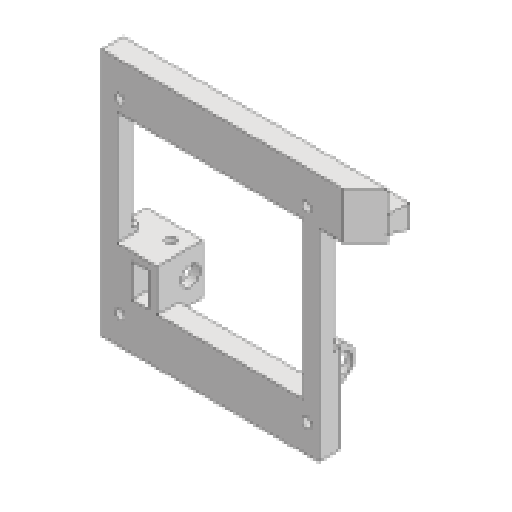
# Autodesk Inventor part: Rail_carriage_y_top_v2
Saved by Autodesk Inventor 2023 (Build 270158000, 158)
## iProperties
Created: 2022-01-11
Part Number: Rail_carriage_y_top_v2
Material: Generic
Document SubType Name: Modeling
Designer: CDT
Density: 1 g/cm^3
Appearance: Default
Author: CDT
Autodesk Inventor part; units mm, degrees
ref_plane "YZ Plane" through (0, 0, 0) normal (1, 0, 0) x (0, 1, 0)
ref_plane "XZ Plane" through (0, 0, 0) normal (0, 1, 0) x (-1, 0, 0)
sketch "Sketch1" plane through (0, 0, 0) normal (0, 0, 1) x (1, 0, 0)
  line L0 (58.7032, 31.1168) -> (-11.2968, 31.1168)
  line L1 (-11.2968, 31.1168) -> (-11.2968, -48.8832)
  line L2 (-11.2968, -48.8832) -> (58.7032, -48.8832)
  line L3 (58.7032, -48.8832) -> (58.7032, 31.1168)
  line L4 (53.7032, 16.1168) -> (-6.2968, 16.1168)
  line L5 (-6.2968, 16.1168) -> (-6.2968, -33.8832)
  line L6 (-6.2968, -33.8832) -> (53.7032, -33.8832)
  line L7 (53.7032, -33.8832) -> (53.7032, 16.1168)
  line L8 (58.7032, 31.1168) -> (73.7032, 31.1168)
  line L9 (73.7032, 31.1168) -> (73.7032, 16.1168)
  line L10 (73.7032, 16.1168) -> (58.7032, 16.1168)
  line L11 (58.7032, 16.1168) -> (58.7032, 31.1168)
  point P0 (0, 0)
  dimension "d0" = 70
  dimension "d1" = 80
  dimension "d4" = 60
  dimension "d5" = 50
  dimension "d6" = 15
  dimension "d7" = 5
  dimension "d76" = 15
  dimension "d77" = 15
  constraints: 24 end point, 6 parallel, 3 horizontal, 3 perpendicular
  measures "d0" distance of L2.end L1.end
  measures "d1" distance of L1.end L0.end
  measures "d4" distance of L6.end L5.end
  measures "d5" distance of L5.end L4.end
  measures "d6" distance between parallel lines of L0 L4
  measures "d7" distance between parallel lines of L3 L7
  measures "d76" distance of L9.end L10.end
  measures "d77" distance of L8.end L9.end
extrude "Extrusion1" add sketch "Sketch1" along normal blind 7
sketch "Sketch2" plane through (0, 0, 0) normal (0, 0, -1) x (-1, 0, 0)
  line L0 (11.2968, 23.8168) -> (-73.7032, 23.8168)
  line L1 (-73.7032, 23.8168) -> (-73.7032, 18.4168)
  line L2 (-73.7032, 18.4168) -> (11.2968, 18.4168)
  line L3 (11.2968, 18.4168) -> (11.2968, 23.8168)
  line L4 (11.2968, 31.1168) -> (11.2968, -48.8832) projected
  line L5 (-58.7032, -48.8832) -> (-58.7032, 16.1168) projected
  line L6 (-73.7032, 16.1168) -> (-73.7032, 31.1168) projected
  line L7 (-73.7032, 31.1168) -> (11.2968, 31.1168) projected
  point P0 (0, 0)
  dimension "d9" = 5.4
  dimension "d10" = 0
  dimension "d78" = 0
  dimension "d79" = 7.3
  constraints: 8 end point, 2 parallel, 1 horizontal, 1 perpendicular
  measures "d9" distance between parallel lines of L2 L0
  measures "d10" distance between parallel lines of L4 L3
  measures "d78" distance between parallel lines of L6 L1
  measures "d79" distance between parallel lines of L7 L0
extrude "Extrusion2" add sketch "Sketch2" along normal blind 5.9 draft 9.9 contours L3 L2 L1 L0
ref_plane "Work Plane1" through (-126.6696, -48.8832, -9) normal (0, 0, 1) x (1, 0, 0)
sketch "Sketch3" plane through (0, 0, 0) normal (0, 0, -1) x (-1, 0, 0)
  line L0 (11.2968, -36.3832) -> (-6.7032, -36.3832)
  line L1 (-6.7032, -36.3832) -> (-6.7032, -20.3832)
  line L2 (-6.7032, -20.3832) -> (11.2968, -20.3832)
  line L3 (11.2968, -20.3832) -> (11.2968, -36.3832)
  line L4 (11.2968, -48.8832) -> (-58.7032, -48.8832) projected
  line L5 (11.2968, 18.4168) -> (11.2968, -48.8832) projected
  line L6 (-55.7032, -33.3832) -> (-53.7032, -33.3832)
  line L7 (-53.7032, -33.3832) -> (-53.7032, -22.3832)
  line L8 (-53.7032, -22.3832) -> (-55.7032, -22.3832)
  line L9 (-55.7032, -22.3832) -> (-55.7032, -33.3832)
  line L10 (-53.7032, -33.8832) -> (6.2968, -33.8832) projected
  line L11 (-53.7032, 16.1168) -> (-53.7032, -33.8832) projected
  point P0 (0, 0)
  point P1 (-54.7032, -33.3832)
  dimension "d14" = 16
  dimension "d15" = 18
  dimension "d16" = 12.5
  dimension "d17" = 0
  dimension "d62" = 11
  dimension "d63" = 0
  dimension "d64" = 2
  dimension "d102" = 0.5
  constraints: 16 end point, 4 parallel, 2 horizontal, 2 perpendicular, 1 midpoint
  measures "d14" distance between parallel lines of L0 L2
  measures "d15" distance between parallel lines of L3 L1
  measures "d16" distance between parallel lines of L4 L0
  measures "d17" distance between parallel lines of L5 L3
  measures "d62" distance between parallel lines of L8 L6
  measures "d63" distance between parallel lines of L11 L7
  measures "d64" distance between parallel lines of L9 L11
  measures "d102" distance from line of L10 point (-54.703, -33.383)
extrude "Extrusion3" add sketch "Sketch3" along normal blind 7.5
sketch "Sketch6" plane through (0, 0, 7) normal (0, 0, 1) x (1, 0, 0)
  line L0 (-6.2968, -20.3832) -> (6.7032, -20.3832) projected
  line L1 (-11.2968, -48.8832) -> (58.7032, -48.8832) projected
  line L2 (6.7032, -20.3832) -> (-11.2968, -20.3832)
  line L3 (-11.2968, -20.3832) -> (-11.2968, -48.8832)
  line L4 (-11.2968, -48.8832) -> (6.7032, -48.8832)
  line L5 (6.7032, -48.8832) -> (6.7032, -20.3832)
  point P0 (0, 0)
  point P1 (6.7032, -48.8832)
  point P2 (-6.2968, -20.3832)
  constraints: 8 end point, 2 parallel, 1 horizontal, 1 perpendicular
extrude "Extrusion6" add sketch "Sketch6" against normal up to surface (7 mm away)
sketch "Sketch9" plane through (-11.2968, -48.8832, 7) normal (-1, 0, 0) x (0, 0, 1)
  circle A0 centre (-10.75, 20.5) radius 3.125
  line L0 (0, 80) -> (0, 0) projected
  line L1 (-7, 0) -> (0, 0) projected
  line L2 (-7, 28.5) -> (-7, 65) projected
  point P0 (-7, 48.8832)
  point P1 (-4, 28.5)
  point P2 (-7, 65)
  dimension "d44" = 6.25
  dimension "d46" = 20.5
  dimension "d65" = 3.75
  constraints: 1 centre point, 1 other
  measures "d44" diameter of A0
  measures "d46" distance from line of L1 A0.centre
extrude "Extrusion8" cut sketch "Sketch9" against normal through all
sketch "Sketch10" plane through (0, 0, -7.5) normal (0, 0, -1) x (-1, 0, 0)
  line L0 (1.4968, -23.0332) -> (-3.7032, -23.0332)
  line L1 (-3.7032, -23.0332) -> (-3.7032, -33.7332)
  line L2 (-3.7032, -33.7332) -> (1.4968, -33.7332)
  line L3 (1.4968, -33.7332) -> (1.4968, -23.0332)
  line L4 (11.2968, -20.3832) -> (-6.7032, -20.3832) projected
  line L5 (-6.7032, -36.3832) -> (11.2968, -36.3832) projected
  line L6 (-6.7032, -20.3832) -> (-6.7032, -36.3832) projected
  point P0 (0, 0)
  dimension "d49" = 5.2
  dimension "d50" = 10.7
  dimension "d51" = 2.65
  dimension "d52" = 2.65
  dimension "d53" = 3
  constraints: 8 end point, 2 parallel, 1 horizontal, 1 perpendicular
  measures "d49" distance between parallel lines of L3 L1
  measures "d50" distance between parallel lines of L2 L0
  measures "d51" distance between parallel lines of L4 L0
  measures "d52" distance between parallel lines of L5 L2
  measures "d53" distance between parallel lines of L6 L1
extrude "Extrusion9" cut sketch "Sketch10" against normal through all
sketch "Sketch11" plane through (-6.2968, -20.3832, 7) normal (0, 1, 0) x (1, 0, 0)
  circle A0 centre (8, 9.5) radius 1.5
  line L0 (10, 14.5) -> (10, 0) projected
  line L1 (-5, 14.5) -> (13, 14.5) projected
  point P0 (6.2968, 7)
  dimension "d56" = 3
  dimension "d57" = 2
  dimension "d58" = 5
  constraints: 1 centre point
  measures "d56" diameter of A0
  measures "d57" distance from line of L0 A0.centre
  measures "d58" distance from line of L1 A0.centre
extrude "Extrusion10" cut sketch "Sketch11" against normal blind 5
sketch "Sketch12" plane through (0, 0, 0) normal (0, 0, -1) x (-1, 0, 0)
  line L0 (-58.7032, -20.3832) -> (-53.7032, -20.3832)
  line L1 (-53.7032, -20.3832) -> (-53.7032, 12.1168)
  line L2 (-53.7032, 12.1168) -> (-58.7032, 12.1168)
  line L3 (-58.7032, 12.1168) -> (-58.7032, -20.3832)
  line L4 (-53.7032, -22.3832) -> (-55.7032, -22.3832) projected
  line L5 (-53.7032, 16.1168) -> (-53.7032, -22.3832) projected
  line L6 (6.2968, 16.1168) -> (-53.7032, 16.1168) projected
  line L7 (-58.7032, -48.8832) -> (-58.7032, 16.1168) projected
  line L8 (6.2968, -18.3832) -> (11.2968, -18.3832)
  line L9 (11.2968, -18.3832) -> (11.2968, 11.1168)
  line L10 (11.2968, 11.1168) -> (6.2968, 11.1168)
  line L11 (6.2968, 11.1168) -> (6.2968, -18.3832)
  line L12 (11.2968, -20.3832) -> (-6.7032, -20.3832) projected
  line L13 (6.2968, -20.3832) -> (6.2968, 16.1168) projected
  line L14 (11.2968, 18.4168) -> (11.2968, -20.3832) projected
  point P0 (0, 0)
  point P1 (-58.7032, 18.2168)
  point P2 (-53.7032, -33.8832)
  dimension "d66" = 2
  dimension "d67" = 0
  dimension "d68" = 4
  dimension "d69" = 0
  dimension "d70" = 2
  dimension "d71" = 0
  dimension "d72" = 0
  dimension "d73" = 5
  constraints: 16 end point, 4 parallel, 2 horizontal, 2 perpendicular
  measures "d66" distance between parallel lines of L4 L0
  measures "d67" distance between parallel lines of L5 L1
  measures "d68" distance between parallel lines of L6 L2
  measures "d69" distance between parallel lines of L7 L3
  measures "d70" distance between parallel lines of L12 L8
  measures "d71" distance between parallel lines of L13 L11
  measures "d72" distance between parallel lines of L14 L9
  measures "d73" distance between parallel lines of L6 L10
extrude "Extrusion11" cut sketch "Sketch12" against normal blind 2.5 contours L3 L2 L1 L0 | L11 L10 L9 L8
sketch "Sketch13" plane through (0, 0, -7.5) normal (0, 0, -1) x (-1, 0, 0)
  line L0 (-55.7032, -22.3832) -> (-55.7032, -33.3832) projected
  line L1 (-53.7032, -22.3832) -> (-55.7032, -22.3832) projected
  line L2 (-55.7032, -33.3832) -> (-53.7032, -33.3832)
  line L3 (-53.7032, -33.3832) -> (-53.7032, -22.3832)
  line L4 (-53.7032, -22.3832) -> (-55.7032, -22.3832)
  line L5 (-55.7032, -22.3832) -> (-55.7032, -33.3832)
  point P0 (0, 0)
  constraints: 8 end point, 2 parallel, 1 horizontal, 1 perpendicular
extrude "Extrusion12" cut sketch "Sketch13" against normal blind 0.5
chamfer "Chamfer1" distance 3 angle 45 2 edges at (54.7032, -22.3832, -7) (54.7032, -33.3832, -7)
sketch "Sketch14" plane through (0, 0, 7) normal (0, 0, 1) x (1, 0, 0)
  circle A0 centre (-5.2968, 20.1168) radius 1.5
  circle A1 centre (54.7032, 20.1168) radius 1.5
  circle A2 centre (-5.2968, -39.8832) radius 1.5
  circle A3 centre (54.7032, -39.8832) radius 1.5
  line L0 (-11.2968, -48.8832) -> (58.7032, -48.8832) projected
  line L1 (58.7032, -48.8832) -> (58.7032, 16.1168) projected
  point P0 (0, 0)
  dimension "d85" = 3
  dimension "d86" = 3
  dimension "d87" = 3
  dimension "d88" = 3
  dimension "d89" = 9
  dimension "d90" = 9
  dimension "d91" = 60
  dimension "d92" = 60
  dimension "d93" = 4
  dimension "d94" = 4
  dimension "d95" = 60
  dimension "d96" = 60
  constraints: 4 centre point
  measures "d85" diameter of A0
  measures "d86" diameter of A1
  measures "d87" diameter of A2
  measures "d88" diameter of A3
  measures "d89" distance from line of L0 A3.centre
  measures "d90" distance from line of L0 A2.centre
  measures "d91" distance of A3.centre A1.centre
  measures "d92" distance of A0.centre A2.centre
  measures "d93" distance from line of L1 A3.centre
  measures "d94" distance from line of L1 A1.centre
  measures "d95" distance of A0.centre A1.centre
  measures "d96" distance of A2.centre A3.centre
extrude "Extrusion13" cut sketch "Sketch14" against normal through all
chamfer "Chamfer2" distance 7 angle 45 1 edges at (73.7032, 23.6168, 7)
equation "\"d6\" = -0.5 * d5 + 0.5 * d1"
equation "\"d70\" = d66"
equation "\"d90\" = d89"
equation "\"d92\" = d91"
equation "\"d94\" = d93"
equation "\"d96\" = d95"
body "Solid1"
